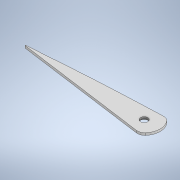
# Autodesk Inventor part: airfoil blueprint
Saved by Autodesk Inventor 2022 (Build 260153000, 153)
## iProperties
Created: 2021-03-06
Part Number: airfoil blueprint
Material: Generic
Document SubType Name: Modeling
Designer: Ferdinand Hubbard
Density: 1 g/cm^3
Appearance: Default
Author: Ferdinand Hubbard
Autodesk Inventor part; units mm, degrees
ref_plane "YZ Plane" through (0, 0, 0) normal (1, 0, 0) x (0, 1, 0)
ref_plane "XZ Plane" through (0, 0, 0) normal (0, 1, 0) x (-1, 0, 0)
ref_plane "XY Plane" through (0, 0, 0) normal (0, 0, 1) x (1, 0, 0)
sketch "Sketch1" plane through (0, 0, 0) normal (0, 1, 0) x (-1, 0, 0)
  arc A0 (210.1622, -7.2025) -> (309.6615, 148.1866) centre (370, 0) ccw construction
  line L0 (370, 0) -> (223.7542, 20.1499)
  circle A1 centre (211.4974, 21.8387) radius 160 construction
  circle A2 centre (369.9872, 0.0018) radius 3 construction
  line L1 (365.7713, 2.7478) -> (370.7713, 2.7478)
  line L2 (370.7713, 2.7478) -> (370.7713, -2.2522)
  line L3 (370.7713, -2.2522) -> (365.7713, -2.2522)
  line L4 (365.7713, -2.2522) -> (365.7713, 2.7478)
  arc A3 (216.7601, 17.6252) -> (215.9023, -5.0762) centre (229.7182, 5.7687) ccw
  circle A4 centre (229.7182, 5.7687) radius 11.5
  circle A5 centre (229.7182, 5.7687) radius 4
  spline S0 degree 4 poles (229.7182, -7.8653) (241.4545, -7.4272) (257.5169, -6.7771) (277.3318, -5.8971) (299.9482, -4.5961) (314.7433, -3.6129) (328.1612, -2.6484) (339.8268, -1.769) (350.012, -1.0496) (357.5866, -0.5225) (364.806, -0.1794) (367.4848, -0.031) (370.1657, -0.0078) (369.9872, 0.0018) knots 0 0 0 0 0 0.270374 0.37387 0.473524 0.56865 0.658428 0.741816 0.817434 0.88334 0.936143 1 1 1 1 1
  arc A6 (223.7542, 20.1499) -> (216.7601, 17.6252) centre (222.6622, 12.2248) ccw
  arc A7 (215.9023, -5.0762) -> (222.4776, -8.1316) centre (222.1952, -0.1366) ccw
  line L5 (222.4776, -8.1316) -> (229.7182, -7.8653)
  point P0 (370, 0)
  point P1 (210.0997, -8.5616)
  point P2 (267.1071, -6.3194)
  point P3 (284.4371, -5.4606)
  point P4 (300.619, -4.5258)
  point P5 (315.5184, -3.5432)
  point P6 (328.988, -2.5786)
  point P7 (340.8625, -1.7041)
  point P8 (350.9622, -0.9861)
  point P9 (359.0984, -0.4682)
  point P10 (365.0855, -0.1602)
  point P11 (368.7597, -0.0285)
  point P12 (368.4073, 0.2194)
  point P13 (365.7713, 0.5826)
  point P14 (220.3414, 20.6201)
  point P15 (365.7713, -0.1283)
  dimension "d5" = 160
  dimension "d25" = 6
  dimension "d26" = 5
  dimension "d27" = 5
  dimension "d41" = 23
  dimension "d60" = 8
  dimension "d65" = 8
  constraints: 12 end point, 9 point on circle, 7 centre point, 3 coincident, 3 tangent, 2 parallel, 2 point on line, 1 equal radius, 1 horizontal, 1 perpendicular, 17 other
  measures "d5" distance of point (211.497, 21.839) L0.start
  measures "d25" diameter of A2
  measures "d26" distance of L2.end L3.end
  measures "d27" distance of L1.end L2.end
  measures "d41" diameter of A4
  measures "d60" diameter of A5
  measures "d65" radius of A6
extrude "Extrusion4" add sketch "Sketch1" along normal blind 2.5 contours S0 L5 A7 A3 A6 L0 L4 | A4
body "Solid4"
